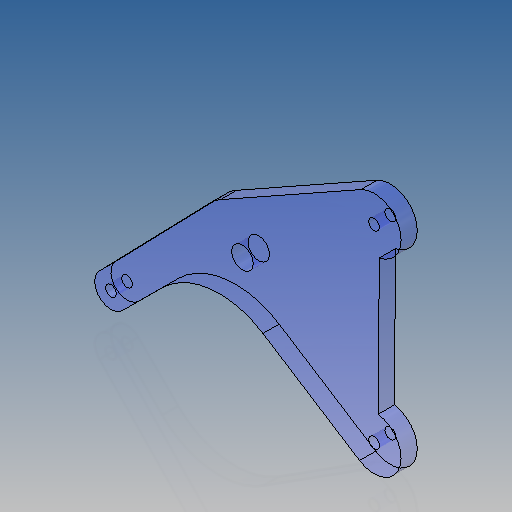
# Autodesk Inventor part: Protector
Saved by Autodesk Inventor 2017 (Build 210142000, 142)
## iProperties
Part Number: Protector
Material: Genérico
Document SubType Name: Modeling
Designer: Leo
Density: 1 g/cm^3
Appearance: Claro - Azul
Author: Leo
Autodesk Inventor part; units mm, degrees
ref_plane "YZ Plane" through (0, 0, 0) normal (1, 0, 0) x (0, 1, 0)
ref_plane "XZ Plane" through (0, 0, 0) normal (0, 1, 0) x (-1, 0, 0)
ref_plane "XY Plane" through (0, 0, 0) normal (0, 0, 1) x (1, 0, 0)
sketch "Boceto1" plane through (0, 0, 0) normal (0, 0, 1) x (1, 0, 0)
  circle A0 centre (23.266, -35) radius 2 projected
  circle A1 centre (120.734, -35) radius 2 projected
  circle A2 centre (120.734, 35) radius 2 projected
  line L0 (18.9572, -30.8245) -> (60.0499, 11.5803)
  line L1 (63.8485, 14.5073) -> (115.8354, 43.718)
  arc A3 (122.658, 25.1868) -> (115.8354, 43.718) centre (120.734, 35) ccw
  line L2 (122.658, 25.1868) -> (122.2685, -25.1184)
  arc A4 (115.3504, -43.4271) -> (122.2685, -25.1184) centre (120.734, -35) ccw
  line L3 (115.3504, -43.4271) -> (79.5564, -20.5604)
  line L4 (42.2427, -24.5784) -> (27.4986, -39.2527)
  arc A5 (18.9572, -30.8245) -> (27.4986, -39.2527) centre (23.266, -35) ccw
  arc A6 (63.8485, 14.5073) -> (60.0499, 11.5803) centre (72, 0) ccw
  circle A7 centre (72, 0) radius 4 projected
  arc A8 (79.5564, -20.5604) -> (42.2427, -24.5784) centre (63.4055, -45.8419) ccw
  point P0 (0, 0)
  point P1 (59.289, -7.6128)
  dimension "d0" = 10
  dimension "d1" = 8
  dimension "d4" = 6
  dimension "d5" = 30
  constraints: 10 end point, 10 point on circle, 9 tangent, 5 centre point, 4 concentric, 2 point on line, 1 equal radius
  measures "d0" radius of A3
  measures "d1" distance edge to line of A3 L2
  measures "d4" radius of A5
  measures "d5" radius of A8
extrude "Extrusión1" add sketch "Boceto1" along normal blind 6
